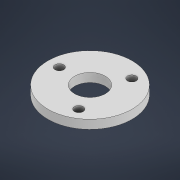
# Autodesk Inventor part: spergear
Saved by Autodesk Inventor 2022 (Build 260153000, 153)
## iProperties
Created: 2021-09-24
Part Number: spergear
Material: 一般
Document SubType Name: Modeling
Designer: shiok
Density: 1 g/cm^3
Appearance: 既定
Author: shiok
Autodesk Inventor part; units mm, degrees
ref_plane "YZ Plane" through (0, 0, 0) normal (1, 0, 0) x (0, 1, 0)
ref_plane "XZ Plane" through (0, 0, 0) normal (0, 1, 0) x (-1, 0, 0)
ref_plane "XY Plane" through (0, 0, 0) normal (0, 0, 1) x (1, 0, 0)
sketch "スケッチ1" plane through (0, 0, 0) normal (0, 1, 0) x (-1, 0, 0)
  circle A0 centre (0, 0) radius 9.6
  circle A1 centre (7, 0) radius 1
  circle A2 centre (-3.5, 6.0622) radius 1
  circle A3 centre (-3.5, -6.0622) radius 1
  circle A4 centre (0, 0) radius 3.5
  dimension "d0" = 19.2
  dimension "d3" = 2
  dimension "d4" = 7
  dimension "d7" = 360
  dimension "d9" = 7
  constraints: 5 centre point, 2 coincident, 1 horizontal alignment, 7 other
  measures "d0" diameter of A0
  measures "d3" diameter of A1
  measures "d4" distance of point (0, 0) A1.centre
  measures "d9" diameter of A4
extrude "押し出し1" add sketch "スケッチ1" along normal blind 2
